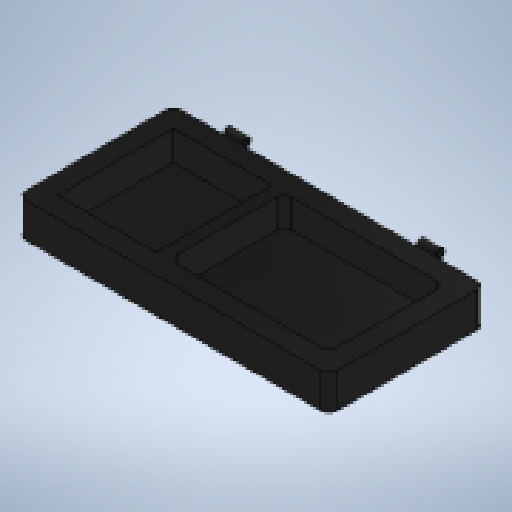
# Autodesk Inventor part: PinecilCaseTop
Saved by Autodesk Inventor 2026 (Build 300175050, 175E)
## iProperties
Created: 2025-10-09
Part Number: PinecilCaseTop
Material: Generic
Document SubType Name: Modeling
Designer: Nicholas M
Density: 1 g/cm^3
Appearance: Smooth - Black
Author: Nicholas M
Autodesk Inventor part; units mm, degrees
ref_plane "YZ Plane" through (0, 0, 0) normal (1, 0, 0) x (0, 1, 0)
sketch "Block1" plane through (0, 0, 0) normal (0, 0, 1) x (1, 0, 0)
  line L0 (-92.3777, -26.6543) -> (-88.0585, -24.932)
  line L1 (-88.0585, -24.932) -> (-90.5223, -30.5169)
  line L2 (-90.5223, -30.5169) -> (-92.3777, -26.6543)
  line L3 (-82.6728, -30.6025) -> (-86.5169, -21.848)
  line L4 (-86.5169, -21.848) -> (-78.7913, -21.848)
  line L5 (-78.7913, -21.848) -> (-82.6728, -30.6025)
  line L6 (-73.749, -30.6978) -> (-70.5333, -23.3906)
  line L7 (-70.5333, -23.3906) -> (-78.2018, -20.0418)
  line L8 (-78.2018, -20.0418) -> (-73.749, -30.6978)
  line L9 (-91.4821, -33.1183) -> (-92.6584, -35.7829)
  line L10 (-92.6584, -35.7829) -> (-96.2473, -32.5216)
  line L11 (-96.2473, -32.5216) -> (-96.2473, -32.5267)
  line L12 (-96.2473, -32.5267) -> (-92.6584, -29.2654)
  line L13 (-92.6584, -29.2654) -> (-91.4738, -31.9484)
  line L14 (-91.4738, -31.9484) -> (-91.406, -32.1157)
  line L15 (-91.406, -32.1157) -> (-91.3738, -32.2216)
  line L16 (-91.3738, -32.2216) -> (-91.3646, -32.723)
  line L17 (-91.3646, -32.723) -> (-91.3835, -32.8054)
  line L18 (-91.3835, -32.8054) -> (-91.4669, -33.0819)
  line L19 (-91.4669, -33.0819) -> (-91.4821, -33.1183)
  line L20 (-92.3777, -38.3926) -> (-88.0585, -40.1159)
  line L21 (-88.0585, -40.1159) -> (-90.5227, -34.5314)
  line L22 (-90.5227, -34.5314) -> (-92.3777, -38.3926)
  line L23 (-83.291, -32.7742) -> (-83.3287, -32.8862)
  line L24 (-83.3287, -32.8862) -> (-86.6061, -40.4026)
  line L25 (-86.6061, -40.4026) -> (-89.89, -32.8687)
  line L26 (-89.89, -32.8687) -> (-89.9241, -32.7724)
  line L27 (-89.9241, -32.7724) -> (-89.9531, -32.5222)
  line L28 (-89.9531, -32.5222) -> (-89.9241, -32.277)
  line L29 (-89.9241, -32.277) -> (-89.89, -32.1807)
  line L30 (-89.89, -32.1807) -> (-86.606, -24.6467)
  line L31 (-86.606, -24.6467) -> (-83.3287, -32.1655)
  line L32 (-83.3287, -32.1655) -> (-83.2946, -32.2628)
  line L33 (-83.2946, -32.2628) -> (-83.2946, -32.2651)
  line L34 (-83.2946, -32.2651) -> (-83.2845, -32.7387)
  line L35 (-83.2845, -32.7387) -> (-83.291, -32.7742)
  line L36 (-82.6728, -34.4458) -> (-86.5169, -43.2003)
  line L37 (-86.5169, -43.2003) -> (-78.7913, -43.2003)
  line L38 (-78.7913, -43.2003) -> (-82.6728, -34.4458)
  line L39 (-73.749, -34.3508) -> (-70.5329, -41.6576)
  line L40 (-70.5329, -41.6576) -> (-78.2014, -45.0065)
  line L41 (-78.2014, -45.0065) -> (-73.749, -34.3508)
  line L42 (-73.1171, -32.5174) -> (-73.0949, -32.6594)
  line L43 (-73.0949, -32.6594) -> (-73.0166, -32.9137)
  line L44 (-73.0166, -32.9137) -> (-69.6871, -40.3822)
  line L45 (-69.6871, -40.3822) -> (-66.6673, -33.544)
  line L46 (-66.6673, -33.544) -> (-66.4005, -33.3699)
  line L47 (-66.4005, -33.3699) -> (-62.4471, -33.3699)
  line L48 (-62.4471, -33.3699) -> (-62.4471, -31.677)
  line L49 (-62.4471, -31.677) -> (-66.4001, -31.677)
  line L50 (-66.4001, -31.677) -> (-66.6668, -31.5028)
  line L51 (-66.6668, -31.5028) -> (-69.6862, -24.6644)
  line L52 (-69.6862, -24.6644) -> (-73.0185, -32.1336)
  line L53 (-73.0185, -32.1336) -> (-73.0969, -32.3879)
  line L54 (-73.0969, -32.3879) -> (-73.1171, -32.5174)
  line L55 (-74.4413, -32.7925) -> (-78.1804, -41.4623)
  line L56 (-78.1804, -41.4623) -> (-81.8914, -32.9206)
  line L57 (-81.8914, -32.9206) -> (-81.8914, -32.1267)
  line L58 (-81.8914, -32.1267) -> (-78.1804, -23.5851)
  line L59 (-78.1804, -23.5851) -> (-74.4413, -32.2548)
  line L60 (-74.4413, -32.2548) -> (-74.3846, -32.4778)
  line L61 (-74.3846, -32.4778) -> (-74.3846, -32.564)
  line L62 (-74.3846, -32.564) -> (-74.4413, -32.7925)
  point P0 (-81.4916, -32.5285)
sketch "Sketch1" plane through (0, 0, 0) normal (0, 1, 0) x (-1, 0, 0)
  line L0 (0, 0) -> (127, 0)
  line L1 (127, 0) -> (127, -63.5)
  line L2 (127, -63.5) -> (0, -63.5)
  line L3 (0, -63.5) -> (0, 0)
  line L4 (123.825, -60.325) -> (123.825, -3.175)
  line L5 (123.825, -3.175) -> (3.175, -3.175)
  line L6 (3.175, -3.175) -> (3.175, -60.325)
  line L7 (3.175, -60.325) -> (123.825, -60.325)
  dimension "d0" = 127
  dimension "d1" = 63.5
  dimension "d2" = 3.175
  constraints: 16 end point, 4 parallel, 2 perpendicular, 1 horizontal, 3 other
  measures "d0" distance of L1.end L2.end
  measures "d1" distance of L2.end L0.start
  measures "d2" distance between parallel lines of L1 L4
extrude "Extrusion1" add sketch "Sketch1" along normal blind 3.175 contours L0 L1 L2 L3 | L7 L6 L5 L4
extrude "Extrusion2" add sketch "Sketch1" along normal blind 17.78
fillet "Fillet1" radius 3.175 8 edges at (0, 8.89, 0) (0, 8.89, -63.5) (-127, 8.89, -63.5) (-127, 8.89, 0) (-123.825, 10.4775, -3.175) (-3.175, 10.4775, -3.175) (-123.825, 10.4775, -60.325) (-3.175, 10.4775, -60.325)
sketch "Sketch6" plane through (0, 0, -3.175) normal (1, 0, 0) x (0, 0, -1)
  line L0 (57.15, 17.78) -> (57.15, 0) projected
  line L1 (0, 17.78) -> (57.15, 17.78) projected
  line L2 (0, 0) -> (0, 17.78) projected
  line L3 (0, 0) -> (57.15, 0) projected
  line L4 (60.325, 17.78) -> (57.15, 17.78) projected
  line L5 (57.15, 17.78) -> (57.15, 0) projected
  line L6 (57.15, 0) -> (60.325, 0) projected
  line L7 (60.325, 0) -> (60.325, 17.78) projected
  circle A0 centre (62.23, 17.78) radius 1.905
  circle A1 centre (62.23, 17.78) radius 0.635
  line L8 (63.577, 16.433) -> (60.325, 13.1809)
  point P0 (-3.175, 0)
  dimension "d53" = 3.81
  dimension "d54" = 1.27
  dimension "d55" = 45
  constraints: 2 centre point, 2 end point, 2 point on circle, 1 coincident, 1 horizontal alignment, 1 point on line, 1 tangent
  measures "d53" diameter of A0
  measures "d54" diameter of A1
  measures "d55" angle of L7 L8
ref_plane "Work Plane7" through (-63.5, 0, -3.175) normal (1, 0, 0) x (0, 0, -1)
ref_plane "Work Plane8" through (-20.32, 0, -3.175) normal (1, 0, 0) x (0, 0, -1)
extrude "Extrusion9" add sketch "Sketch6" against normal blind 7.62 from surface at -20.32 contours A0 L8 L7 | A0
mirror "Mirror3" about plane through (-63.5, 0, -3.175) normal (1, 0, 0) of "Extrusion9"
sketch "Sketch7" plane through (0, 0, 0) normal (0, -1, 0) x (1, 0, 0)
  line L0 (-127, -60.325) -> (-127, -3.175) projected
  line L1 (0, -3.175) -> (0, -60.325) projected
  arc A0 (-123.825, 0) -> (-127, -3.175) centre (-123.825, -3.175) ccw projected
  line L2 (-127, -60.325) -> (-127, -3.175) projected
  arc A1 (-127, -60.325) -> (-123.825, -63.5) centre (-123.825, -60.325) ccw projected
  line L3 (-3.175, -63.5) -> (-123.825, -63.5) projected
  arc A2 (-3.175, -63.5) -> (0, -60.325) centre (-3.175, -60.325) ccw projected
  line L4 (0, -3.175) -> (0, -60.325) projected
  arc A3 (0, -3.175) -> (-3.175, 0) centre (-3.175, -3.175) ccw projected
  line L5 (-123.825, 0) -> (-3.175, 0) projected
  line L6 (-99.7806, -25.8809) -> (-95.4614, -24.1586)
  line L7 (-95.4614, -24.1586) -> (-97.9251, -29.7435)
  line L8 (-97.9251, -29.7435) -> (-99.7806, -25.8809)
  line L9 (-90.0756, -29.8291) -> (-93.9198, -21.0746)
  line L10 (-93.9198, -21.0746) -> (-86.1942, -21.0746)
  line L11 (-86.1942, -21.0746) -> (-90.0756, -29.8291)
  line L12 (-81.1519, -29.9244) -> (-77.9362, -22.6172)
  line L13 (-77.9362, -22.6172) -> (-85.6047, -19.2683)
  line L14 (-85.6047, -19.2683) -> (-81.1519, -29.9244)
  line L15 (-98.8849, -32.3449) -> (-100.0613, -35.0095)
  line L16 (-100.0613, -35.0095) -> (-103.6502, -31.7482)
  line L17 (-103.6502, -31.7482) -> (-103.6502, -31.7533)
  line L18 (-103.6502, -31.7533) -> (-100.0613, -28.492)
  line L19 (-100.0613, -28.492) -> (-98.8767, -31.175)
  line L20 (-98.8767, -31.175) -> (-98.8089, -31.3423)
  line L21 (-98.8089, -31.3423) -> (-98.7767, -31.4482)
  line L22 (-98.7767, -31.4482) -> (-98.7675, -31.9495)
  line L23 (-98.7675, -31.9495) -> (-98.7863, -32.032)
  line L24 (-98.7863, -32.032) -> (-98.8697, -32.3085)
  line L25 (-98.8697, -32.3085) -> (-98.8849, -32.3449)
  line L26 (-99.7806, -37.6192) -> (-95.4614, -39.3424)
  line L27 (-95.4614, -39.3424) -> (-97.9256, -33.758)
  line L28 (-97.9256, -33.758) -> (-99.7806, -37.6192)
  line L29 (-90.6938, -32.0008) -> (-90.7316, -32.1128)
  line L30 (-90.7316, -32.1128) -> (-94.009, -39.6292)
  line L31 (-94.009, -39.6292) -> (-97.2929, -32.0953)
  line L32 (-97.2929, -32.0953) -> (-97.327, -31.9989)
  line L33 (-97.327, -31.9989) -> (-97.356, -31.7488)
  line L34 (-97.356, -31.7488) -> (-97.327, -31.5036)
  line L35 (-97.327, -31.5036) -> (-97.2929, -31.4073)
  line L36 (-97.2929, -31.4073) -> (-94.0089, -23.8733)
  line L37 (-94.0089, -23.8733) -> (-90.7316, -31.3921)
  line L38 (-90.7316, -31.3921) -> (-90.6975, -31.4893)
  line L39 (-90.6975, -31.4893) -> (-90.6975, -31.4917)
  line L40 (-90.6975, -31.4917) -> (-90.6874, -31.9653)
  line L41 (-90.6874, -31.9653) -> (-90.6938, -32.0008)
  line L42 (-90.0756, -33.6723) -> (-93.9198, -42.4268)
  line L43 (-93.9198, -42.4268) -> (-86.1942, -42.4268)
  line L44 (-86.1942, -42.4268) -> (-90.0756, -33.6723)
  line L45 (-81.1519, -33.5774) -> (-77.9357, -40.8842)
  line L46 (-77.9357, -40.8842) -> (-85.6042, -44.233)
  line L47 (-85.6042, -44.233) -> (-81.1519, -33.5774)
  line L48 (-80.52, -31.744) -> (-80.4978, -31.886)
  line L49 (-80.4978, -31.886) -> (-80.4195, -32.1403)
  line L50 (-80.4195, -32.1403) -> (-77.09, -39.6088)
  line L51 (-77.09, -39.6088) -> (-74.0701, -32.7706)
  line L52 (-74.0701, -32.7706) -> (-73.8034, -32.5965)
  line L53 (-73.8034, -32.5965) -> (-69.85, -32.5965)
  line L54 (-69.85, -32.5965) -> (-69.85, -30.9035)
  line L55 (-69.85, -30.9035) -> (-73.8029, -30.9035)
  line L56 (-73.8029, -30.9035) -> (-74.0697, -30.7294)
  line L57 (-74.0697, -30.7294) -> (-77.089, -23.891)
  line L58 (-77.089, -23.891) -> (-80.4214, -31.3601)
  line L59 (-80.4214, -31.3601) -> (-80.4997, -31.6145)
  line L60 (-80.4997, -31.6145) -> (-80.52, -31.744)
  line L61 (-81.8442, -32.0191) -> (-85.5833, -40.6889)
  line L62 (-85.5833, -40.6889) -> (-89.2943, -32.1472)
  line L63 (-89.2943, -32.1472) -> (-89.2943, -31.3533)
  line L64 (-89.2943, -31.3533) -> (-85.5833, -22.8117)
  line L65 (-85.5833, -22.8117) -> (-81.8442, -31.4814)
  line L66 (-81.8442, -31.4814) -> (-81.7875, -31.7044)
  line L67 (-81.7875, -31.7044) -> (-81.7875, -31.7906)
  line L68 (-81.7875, -31.7906) -> (-81.8442, -32.0191)
  point P0 (-69.85, -31.75)
  point P1 (-127, -31.75)
  point P2 (-103.6474, -31.7507)
  dimension "d65" = 69.85
  constraints: 1 horizontal alignment, 1 midpoint, 1 other
extrude "Extrusion10" cut sketch "Sketch7" against normal blind 1.5875 contours L6 L7 L8 | L9 L10 L11 | L14 L13 L12 | L15 L16 L18 L19 L20 L21 L22 L23 L24 L25 | L28 L27 L26 | L29 L30 L31 L32 L33 L34 L35 L36 L37 L38 L39 L40 L41 | L44 L43 L42 | L45 L46 L47 | L60 L59 L58 L57 L56 L55 L54 L53 L52 L51 L50 L49 L48 | L61 L62 L63 L64 L65 L66 L67 L68
sketch "Sketch9" plane through (0, 0, 0) normal (0, -1, 0) x (1, 0, 0)
  line L0 (-81.1519, -33.5774) -> (-77.9357, -40.8842) projected
  line L1 (-77.9357, -40.8842) -> (-85.6042, -44.233) projected
  line L2 (-85.6042, -44.233) -> (-81.1519, -33.5774) projected
  line L3 (-90.0756, -33.6723) -> (-86.1942, -42.4268) projected
  line L4 (-86.1942, -42.4268) -> (-93.9198, -42.4268) projected
  line L5 (-93.9198, -42.4268) -> (-90.0756, -33.6723) projected
  line L6 (-99.7806, -25.8809) -> (-95.4614, -24.1586) projected
  line L7 (-95.4614, -24.1586) -> (-97.9251, -29.7435) projected
  line L8 (-97.9251, -29.7435) -> (-99.7806, -25.8809) projected
  line L9 (-90.6975, -31.4917) -> (-90.6874, -31.9653) projected
  line L10 (-90.6874, -31.9653) -> (-90.6938, -32.0008) projected
  line L11 (-90.6938, -32.0008) -> (-90.7316, -32.1128) projected
  line L12 (-90.7316, -32.1128) -> (-94.009, -39.6292) projected
  line L13 (-94.009, -39.6292) -> (-97.2929, -32.0953) projected
  line L14 (-97.2929, -32.0953) -> (-97.327, -31.9989) projected
  line L15 (-97.327, -31.9989) -> (-97.356, -31.7488) projected
  line L16 (-97.356, -31.7488) -> (-97.327, -31.5036) projected
  line L17 (-97.327, -31.5036) -> (-97.2929, -31.4073) projected
  line L18 (-97.2929, -31.4073) -> (-94.0089, -23.8733) projected
  line L19 (-94.0089, -23.8733) -> (-90.7316, -31.3921) projected
  line L20 (-90.7316, -31.3921) -> (-90.6975, -31.4893) projected
  line L21 (-90.6975, -31.4893) -> (-90.6975, -31.4917) projected
  line L22 (-81.8442, -31.4814) -> (-81.7875, -31.7044) projected
  line L23 (-81.7875, -31.7044) -> (-81.7875, -31.7906) projected
  line L24 (-81.7875, -31.7906) -> (-81.8442, -32.0191) projected
  line L25 (-81.8442, -32.0191) -> (-85.5833, -40.6889) projected
  line L26 (-85.5833, -40.6889) -> (-89.2943, -32.1472) projected
  line L27 (-89.2943, -32.1472) -> (-89.2943, -31.3533) projected
  line L28 (-89.2943, -31.3533) -> (-85.5833, -22.8117) projected
  line L29 (-85.5833, -22.8117) -> (-81.8442, -31.4814) projected
  line L30 (-81.1519, -29.9244) -> (-85.6047, -19.2683) projected
  line L31 (-85.6047, -19.2683) -> (-77.9362, -22.6172) projected
  line L32 (-77.9362, -22.6172) -> (-81.1519, -29.9244) projected
  line L33 (-99.7806, -37.6192) -> (-97.9256, -33.758) projected
  line L34 (-97.9256, -33.758) -> (-95.4614, -39.3424) projected
  line L35 (-95.4614, -39.3424) -> (-99.7806, -37.6192) projected
  line L36 (-98.7863, -32.032) -> (-98.8697, -32.3085) projected
  line L37 (-98.8697, -32.3085) -> (-98.8849, -32.3449) projected
  line L38 (-98.8849, -32.3449) -> (-100.0613, -35.0095) projected
  line L39 (-100.0613, -35.0095) -> (-103.6474, -31.7507) projected
  line L40 (-103.6474, -31.7507) -> (-100.0613, -28.492) projected
  line L41 (-100.0613, -28.492) -> (-98.8767, -31.175) projected
  line L42 (-98.8767, -31.175) -> (-98.8089, -31.3423) projected
  line L43 (-98.8089, -31.3423) -> (-98.7767, -31.4482) projected
  line L44 (-98.7767, -31.4482) -> (-98.7675, -31.9495) projected
  line L45 (-98.7675, -31.9495) -> (-98.7863, -32.032) projected
  line L46 (-90.0756, -29.8291) -> (-93.9198, -21.0746) projected
  line L47 (-93.9198, -21.0746) -> (-86.1942, -21.0746) projected
  line L48 (-86.1942, -21.0746) -> (-90.0756, -29.8291) projected
  line L49 (-80.4978, -31.886) -> (-80.52, -31.744) projected
  line L50 (-80.52, -31.744) -> (-80.4997, -31.6145) projected
  line L51 (-80.4997, -31.6145) -> (-80.4214, -31.3601) projected
  line L52 (-80.4214, -31.3601) -> (-77.089, -23.891) projected
  line L53 (-77.089, -23.891) -> (-74.0697, -30.7294) projected
  line L54 (-74.0697, -30.7294) -> (-73.8029, -30.9035) projected
  line L55 (-73.8029, -30.9035) -> (-69.85, -30.9035) projected
  line L56 (-69.85, -30.9035) -> (-69.85, -32.5965) projected
  line L57 (-69.85, -32.5965) -> (-73.8034, -32.5965) projected
  line L58 (-73.8034, -32.5965) -> (-74.0701, -32.7706) projected
  line L59 (-74.0701, -32.7706) -> (-77.09, -39.6088) projected
  line L60 (-77.09, -39.6088) -> (-80.4195, -32.1403) projected
  line L61 (-80.4195, -32.1403) -> (-80.4978, -31.886) projected
  arc A0 (-123.825, 0) -> (-127, -3.175) centre (-123.825, -3.175) ccw projected
  line L62 (-127, -60.325) -> (-127, -3.175) projected
  arc A1 (-127, -60.325) -> (-123.825, -63.5) centre (-123.825, -60.325) ccw projected
  line L63 (-3.175, -63.5) -> (-123.825, -63.5) projected
  arc A2 (-3.175, -63.5) -> (0, -60.325) centre (-3.175, -60.325) ccw projected
  line L64 (0, -3.175) -> (0, -60.325) projected
  arc A3 (0, -3.175) -> (-3.175, 0) centre (-3.175, -3.175) ccw projected
  line L65 (-123.825, 0) -> (-3.175, 0) projected
  arc A4 (-3.175, -61.595) -> (-1.905, -60.325) centre (-3.175, -60.325) ccw
  line L66 (-3.175, -61.595) -> (-123.825, -61.595)
  arc A5 (-125.095, -60.325) -> (-123.825, -61.595) centre (-123.825, -60.325) ccw
  line L67 (-125.095, -60.325) -> (-125.095, -3.175)
  arc A6 (-123.825, -1.905) -> (-125.095, -3.175) centre (-123.825, -3.175) ccw
  line L68 (-123.825, -1.905) -> (-3.175, -1.905)
  arc A7 (-1.905, -3.175) -> (-3.175, -1.905) centre (-3.175, -3.175) ccw
  line L69 (-1.905, -3.175) -> (-1.905, -60.325)
  line L70 (-3.81, -59.69) -> (-123.19, -59.69)
  line L71 (-123.19, -59.69) -> (-123.19, -3.81)
  line L72 (-123.19, -3.81) -> (-3.81, -3.81)
  line L73 (-3.81, -3.81) -> (-3.81, -59.69)
  arc A8 (-3.175, -62.5475) -> (-0.9525, -60.325) centre (-3.175, -60.325) ccw
  line L74 (-3.175, -62.5475) -> (-123.825, -62.5475)
  arc A9 (-126.0475, -60.325) -> (-123.825, -62.5475) centre (-123.825, -60.325) ccw
  line L75 (-126.0475, -60.325) -> (-126.0475, -3.175)
  arc A10 (-123.825, -0.9525) -> (-126.0475, -3.175) centre (-123.825, -3.175) ccw
  line L76 (-123.825, -0.9525) -> (-3.175, -0.9525)
  arc A11 (-0.9525, -3.175) -> (-3.175, -0.9525) centre (-3.175, -3.175) ccw
  line L77 (-0.9525, -3.175) -> (-0.9525, -60.325)
  point P0 (0, 0)
  dimension "d74" = 1.905
  dimension "d75" = 1.905
  dimension "d78" = 0.9525
  constraints: 24 end point, 16 point on circle, 8 centre point, 17 other
  measures "d74" distance between parallel lines of L64 L69
  measures "d75" distance between parallel lines of L69 L73
  measures "d78" distance between parallel lines of L64 L77
extrude "Extrusion13" cut sketch "Sketch9" against normal blind 1.5875 contours L65 A3 L64 A2 L63 A1 L62 A0 | L74 A9 L75 A10 L76 A11 L77 A8
sketch "Sketch10" plane through (0, 3.175, 0) normal (0, 1, 0) x (1, 0, 0)
  line L0 (-118.75, 8.25) -> (-78.75, 8.25)
  line L1 (-78.75, 8.25) -> (-78.75, 55.25)
  line L2 (-78.75, 55.25) -> (-118.75, 55.25)
  line L3 (-118.75, 55.25) -> (-118.75, 8.25)
  line L4 (-123.825, 6.35) -> (-123.825, 57.15) projected
  line L5 (-6.35, 3.175) -> (-120.65, 3.175) projected
  line L6 (-3.175, 57.15) -> (-3.175, 6.35) projected
  line L7 (-123.825, 3.175) -> (-123.825, 60.325)
  line L8 (-6.35, 60.325) -> (-120.65, 60.325) projected
  arc A0 (-3.175, 57.15) -> (-6.35, 60.325) centre (-6.35, 57.15) ccw projected
  line L9 (-6.35, 60.325) -> (-120.65, 60.325) projected
  arc A1 (-120.65, 60.325) -> (-123.825, 57.15) centre (-120.65, 57.15) ccw projected
  line L10 (-123.825, 57.15) -> (-123.825, 6.35) projected
  arc A2 (-123.825, 6.35) -> (-120.65, 3.175) centre (-120.65, 6.35) ccw projected
  line L11 (-120.65, 3.175) -> (-6.35, 3.175) projected
  arc A3 (-6.35, 3.175) -> (-3.175, 6.35) centre (-6.35, 6.35) ccw projected
  line L12 (-3.175, 6.35) -> (-3.175, 57.15) projected
  line L13 (-118.877, 8.123) -> (-78.623, 8.123)
  line L14 (-78.623, 8.123) -> (-78.623, 55.377)
  line L15 (-78.623, 55.377) -> (-118.877, 55.377)
  line L16 (-118.877, 55.377) -> (-118.877, 8.123)
  line L17 (-73.548, 3.175) -> (-73.548, 60.325)
  line L18 (-73.548, 8.25) -> (-8.255, 8.25)
  line L19 (-8.255, 8.25) -> (-8.255, 55.25)
  line L20 (-8.255, 55.25) -> (-73.548, 55.25)
  line L21 (-73.548, 55.25) -> (-73.548, 8.25)
  point P0 (0, 0)
  point P1 (-118.75, 31.75)
  point P2 (-123.825, 31.75)
  dimension "d79" = 40
  dimension "d80" = 47
  dimension "d81" = 5.075
  dimension "d83" = 5.075
  dimension "d84" = 0.127
  dimension "d89" = 5.075
  dimension "d91" = 5.08
  constraints: 28 end point, 6 parallel, 5 point on line, 4 perpendicular, 3 collinear, 2 horizontal, 2 midpoint, 1 horizontal alignment, 1 vertical, 3 other
  measures "d79" distance of L2.end L1.end
  measures "d80" distance of L1.end L0.end
  measures "d81" distance between parallel lines of L5 L0
  measures "d83" distance between parallel lines of L3 L7
  measures "d84" distance between parallel lines of L3 L16
  measures "d89" distance between parallel lines of L14 L17
  measures "d91" distance between parallel lines of L6 L19
extrude "Extrusion15" add sketch "Sketch10" along normal up to surface (14.605 mm away) contours L4 A1 L8 L17 L5 A2 | L17 L18 L19 L20 L8 A0 L6 A3 L5
fillet "Fillet5" radius 3.175 4 edges at (-73.548, 10.4775, -8.25) (-73.548, 10.4775, -55.25) (-8.255, 10.4775, -8.25) (-8.255, 10.4775, -55.25)
sketch "Sketch11" plane through (0, 17.78, 0) normal (0, 1, 0) x (1, 0, 0)
  circle A0 centre (-5.08, 5.08) radius 2.54
  line L0 (0, 3.175) -> (0, 60.325) projected
  line L1 (-123.825, 0) -> (-3.175, 0) projected
  line L2 (0, 31.75) -> (-127, 31.75) construction
  line L3 (-127, 60.325) -> (-127, 3.175) projected
  line L4 (-123.825, 0) -> (-3.175, 0) projected
  line L5 (-63.5, 0) -> (-63.5, 63.5) construction
  line L6 (-27.94, 63.5) -> (-99.06, 63.5) projected
  circle A1 centre (-121.92, 5.08) radius 2.54
  circle A2 centre (-5.08, 58.42) radius 2.54
  circle A3 centre (-121.92, 58.42) radius 2.54
  point P0 (0, 0)
  dimension "d92" = 5.08
  dimension "d93" = 5.08
  dimension "d94" = 5.08
  constraints: 4 centre point, 4 end point, 4 midpoint, 3 symmetric about line, 3 other
  measures "d92" diameter of A0
  measures "d93" distance from line of L0 A0.centre
  measures "d94" distance from line of L1 A0.centre
extrude "Extrusion16" cut sketch "Sketch11" against normal blind 3
equation "\"d83\" = d81"
equation "\"d89\" = d81"
body "Solid1"
